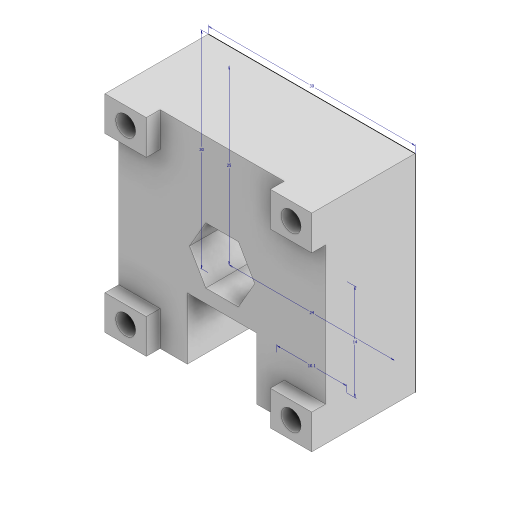
# Autodesk Inventor part: front_door-webcam(FIT0701)-mount
Saved by Autodesk Inventor 2023 (Build 270158000, 158)
## iProperties
Created: 2024-07-08
Part Number: front_door-webcam(FIT0701)-mount
Material: Generic
Document SubType Name: Modeling
Designer: N.Vladimirov
Density: 1 g/cm^3
Appearance: Default
Author: N.Vladimirov
Autodesk Inventor part; units mm, degrees
ref_plane "YZ Plane" through (0, 0, 0) normal (1, 0, 0) x (0, 1, 0)
ref_plane "XZ Plane" through (0, 0, 0) normal (0, 1, 0) x (-1, 0, 0)
ref_plane "XY Plane" through (0, 0, 0) normal (0, 0, 1) x (1, 0, 0)
sketch "Sketch1" plane through (0, 0, 0) normal (0, 0, 1) x (1, 0, 0)
  line L0 (-15, -15) -> (-15, 15)
  line L1 (-15, 15) -> (15, 15)
  line L2 (15, 15) -> (15, -15)
  line L3 (15, -15) -> (-15, 15) construction
  line L4 (-15, -15) -> (15, 15) construction
  line L5 (0, 0) -> (8.0802, 0) construction
  line L6 (0, 0) -> (0, 7.2946) construction
  line L7 (-5.05, -20.05) -> (5.05, -20.05)
  line L8 (5.05, -20.05) -> (5.05, -6.05)
  line L9 (5.05, -6.05) -> (-5.05, -6.05)
  line L10 (-5.05, -6.05) -> (-5.05, -20.05)
  line L11 (-5.05, -20.05) -> (5.05, -6.05) construction
  line L12 (5.05, -20.05) -> (-5.05, -6.05) construction
  line L13 (15, -15) -> (5.05, -15)
  line L14 (-5.05, -15) -> (-15, -15)
  point P0 (-12, -12.5)
  point P1 (12, -12.5)
  point P2 (-12, 12.5)
  point P3 (12, 12.5)
  point P4 (0, -13.05)
  dimension "d0" = 30
  dimension "d1" = 30
  dimension "d4" = 24
  dimension "d7" = 25
  dimension "d10" = 10.1
  dimension "d11" = 14
  constraints: 30 end point, 5 parallel, 4 horizontal, 3 midpoint, 3 perpendicular, 2 point on line, 2 symmetric about line, 2 vertical, 3 other
  measures "d0" distance of L0.end L1.end
  measures "d1" distance of L0.start L0.end
  measures "d4" distance of point (-12, -12.5) point (12, -12.5)
  measures "d7" distance of point (-12, -12.5) point (-12, 12.5)
  measures "d10" distance of L7.start L7.end
  measures "d11" distance of L8.end L7.end
extrude "Extrusion1" add sketch "Sketch1" along normal blind 15 contours L0 L1 L2 L13 L8 L9 L10 L14
hole "Hole1" at (12, 12.5, 0) at (-12, 12.5, 0) at (-12, -12.5, 0) at (12, -12.5, 0) direction (0, 0, 1) diameter 2.9 end through all
sketch "Sketch2" plane through (0, 0, 0) normal (0, 0, -1) x (-1, 0, 0)
  point P0 (0, 0)
  point P1 (0, 0)
  constraints: 1 coincident
hole "Hole2" at (0, 0, 0) direction (0, 0, 1) diameter 5.3 end through all clearance for "Flat Head Machine Screw" size "M5" standard "Ansi Metric M Profile"
sketch "Sketch3" plane through (0, 0, 15) normal (0, 0, 1) x (1, 0, 0)
  line L0 (15, 15) -> (-15, 15) projected
  line L1 (-15, 15) -> (-9, 15)
  line L2 (-9, 15) -> (-9, 10)
  line L3 (-9, 10) -> (-15, 10)
  line L4 (-15, 10) -> (-15, 15)
  line L5 (15, -15) -> (15, 15) projected
  line L6 (15, 15) -> (9, 15)
  line L7 (9, 15) -> (9, 10)
  line L8 (9, 10) -> (15, 10)
  line L9 (15, 10) -> (15, 15)
  line L10 (-15, -15) -> (-5.05, -15) projected
  line L11 (-15, -15) -> (-9, -15)
  line L12 (-9, -15) -> (-9, -10)
  line L13 (-9, -10) -> (-15, -10)
  line L14 (-15, -10) -> (-15, -15)
  line L15 (15, -15) -> (9, -15)
  line L16 (9, -15) -> (9, -10)
  line L17 (9, -10) -> (15, -10)
  line L18 (15, -10) -> (15, -15)
  circle A0 centre (0, 0) radius 2.65 projected
  circle A1 centre (-12, -12.5) radius 1.45 projected
  circle A2 centre (12, 12.5) radius 1.45 projected
  circle A3 centre (-12, 12.5) radius 1.45 projected
  circle A4 centre (12, -12.5) radius 1.45 projected
  line L19 (15, 15) -> (-15, 15) projected
  line L20 (-15, 15) -> (-15, -15) projected
  line L21 (-15, -15) -> (-5.05, -15) projected
  line L22 (-5.05, -15) -> (-5.05, -6.05) projected
  line L23 (-5.05, -6.05) -> (5.05, -6.05) projected
  line L24 (5.05, -6.05) -> (5.05, -15) projected
  line L25 (5.05, -15) -> (15, -15) projected
  line L26 (15, -15) -> (15, 15) projected
  dimension "d28" = 6
  dimension "d29" = 5
  dimension "d30" = 6
  dimension "d31" = 5
  dimension "d32" = 6
  dimension "d33" = 5
  constraints: 32 end point, 8 parallel, 4 horizontal, 4 perpendicular, 4 point on line
  measures "d28" distance of L2.end L3.end
  measures "d29" distance of L1.end L2.end
  measures "d30" distance of L8.end L7.end
  measures "d31" distance of L7.end L6.end
  measures "d32" distance of L13.end L12.end
  measures "d33" distance of L12.end L11.end
extrude "Extrusion2" cut sketch "Sketch3" against normal blind 2 contours L7 L8 L5 L17 L16 L25 L24 L23 L22 L10 L12 L13 L20 L3 L2 L0
sketch "Sketch4" plane through (0, 0, 13) normal (0, 0, 1) x (1, 0, 0)
  line L0 (2.3671, 4.1) -> (4.7343, 0)
  line L1 (4.7343, 0) -> (2.3671, -4.1)
  line L2 (2.3671, -4.1) -> (-2.3671, -4.1)
  line L3 (-2.3671, -4.1) -> (-4.7343, 0)
  line L4 (-4.7343, 0) -> (-2.3671, 4.1)
  line L5 (-2.3671, 4.1) -> (2.3671, 4.1)
  point P0 (0, 0)
  point P1 (0, 0)
  dimension "d36" = 8.2
  constraints: 12 end point, 1 coincident, 13 other
  measures "d36" distance between parallel lines of L2 L5
extrude "Extrusion3" cut sketch "Sketch4" against normal blind 10
body "Solid1"
